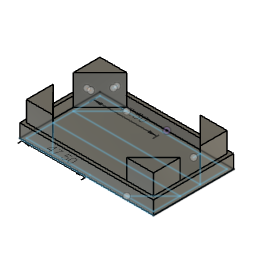
ex62 (Autodesk Fusion 360 design; units mm, degrees)
Autodesk Fusion 360 part; units mm, degrees
sketch "Sketch1" plane through (0, 0, 0) normal (0, 0, 1) x (1, 0, 0)
  line L0 (0, 0) -> (50, 0)
  line L1 (0, 0) -> (-50, 0)
  line L2 (0, -60) -> (50, -60)
  line L3 (0, -60) -> (-50, -60)
  line L4 (0, -2.5) -> (47.5, -2.5)
  line L5 (0, -2.5) -> (-47.5, -2.5)
  line L6 (0, -57.5) -> (47.5, -57.5)
  line L7 (0, -57.5) -> (-47.5, -57.5)
  line L8 (-47.5, -2.5) -> (-47.5, -57.5)
  line L9 (47.5, -2.5) -> (47.5, -57.5)
  line L10 (50, -60) -> (50, 0)
  line L11 (-50, -60) -> (-50, 0)
  line L12 (-54.3467, -2.5) -> (-57.3288, -2.5) construction
  line L13 (-47.5, -22.5) -> (47.5, -22.5)
  line L14 (-47.5, 10.1561) -> (-47.5, 7.5248)
  line L15 (-47.5, -22.5) -> (-27.5, -2.5)
  line L16 (27.5, -2.5) -> (27.5, -7.3859)
  line L17 (47.5, -22.5) -> (27.5, -2.5)
  line L18 (-47.5, -37.5) -> (-27.9827, -57.5)
  line L19 (47.5, -37.5) -> (-47.5, -37.5)
  line L20 (27.5, -57.5) -> (47.5, -37.5)
  dimension "d1" = 50
  dimension "d2" = 50
  dimension "d3" = 60
  dimension "d4" = 50
  dimension "d5" = 50
  dimension "d6" = 2.5
  dimension "d7" = 47.5
  dimension "d8" = 47.5
  dimension "d9" = 2.5
  dimension "d10" = 47.5
  dimension "d11" = 47.5
  constraint coincident L0.start L1.start
  constraint horizontal L0
  constraint parallel L0 L1
  constraint perpendicular L7 L8
  constraint perpendicular L6 L9
  constraint perpendicular L0 L10
  constraint perpendicular L1 L11
  constraint perpendicular L11 L19
  constraint perpendicular L1 L14
  constraint coincident L8 L13.start
  constraint coincident L5 L15.end
  constraint perpendicular L4 L16
  constraint coincident L4 L16.start
  constraint coincident L9 L13.end
  constraint coincident L8 L18.start
  constraint coincident L7 L18.end
  constraint coincident L6 L20.start
  constraint coincident L9 L19.start
  measures "d1" distance of L0.start L0.end
  measures "d2" distance of L0.start L1.end
  measures "d3" distance of L0.start L2.start
  measures "d4" distance of L2.start L2.end
  measures "d5" distance of L2.start L3.end
  measures "d6" distance of L0.start L4.start
  measures "d7" distance of L4.start L4.end
  measures "d8" distance of L4.start L5.end
  measures "d9" distance of L2.start L6.start
  measures "d10" distance of L6.start L6.end
  measures "d11" distance of L6.start L7.end
extrude "Extrude1" add sketch "Sketch1" along normal blind 10
extrude "Extrude2" add sketch "Sketch1" along normal blind 25 contours L4 L9 L17 | L5 L8 L15 | L6 L9 L20 | L7 L8 L18
extrude "Extrude3" add sketch "Sketch1" along normal blind 2.5 contours L4 L5 L13 L15 L17 | L8 L9 L13 L19 | L6 L7 L18 L19 L20
